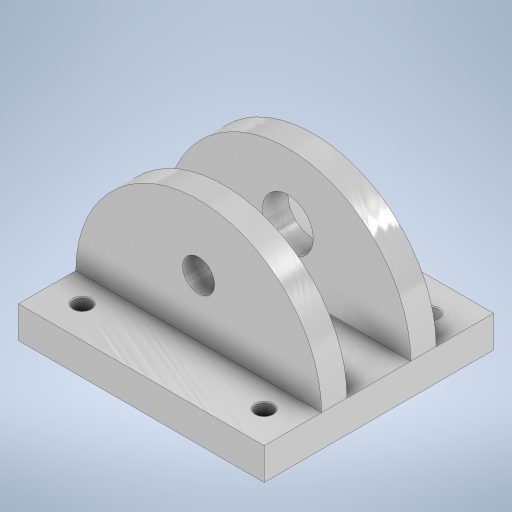
# Autodesk Inventor part: Carriage Top
Saved by Autodesk Inventor 2023 (Build 270158000, 158)
## iProperties
Created: 2023-02-13
Part Number: Carriage Top
Material: Aluminum 6061
Document SubType Name: Modeling
Designer: mbear
Density: 2.7 g/cm^3
Appearance: Machined - Aluminum
Author: mbear
Autodesk Inventor part; units mm, degrees
ref_plane "YZ Plane" through (0, 0, 0) normal (1, 0, 0) x (0, 1, 0)
sketch "Sketch1" plane through (0, 0, 0) normal (0, 1, 0) x (-1, 0, 0)
  line L0 (0, 0) -> (-48.9966, 0)
  line L1 (-48.9966, 0) -> (-48.9966, -45.72)
  line L2 (-48.9966, -45.72) -> (0, -45.72)
  line L3 (0, -45.72) -> (0, 0)
  dimension "d0" = 48.9966
  dimension "d1" = 45.72
  constraints: 8 end point, 2 parallel, 1 horizontal, 1 perpendicular
  measures "d0" distance between parallel lines of L1 L3
  measures "d1" distance between parallel lines of L0 L2
extrude "Extrusion1" add sketch "Sketch1" along normal blind 6.35
sketch "Sketch3" plane through (0, 6.35, 0) normal (0, 1, 0) x (1, 0, 0)
  line L0 (0, 45.72) -> (0, 0) projected
  line L1 (48.9966, 0) -> (48.9966, 45.72) projected
  line L2 (0, 29.21) -> (48.9966, 29.21)
  line L3 (48.9966, 29.21) -> (48.9966, 16.51)
  line L4 (48.9966, 16.51) -> (0, 16.51)
  line L5 (0, 16.51) -> (0, 29.21)
  line L6 (48.9966, 45.72) -> (0, 45.72) projected
  dimension "d4" = 12.7
  dimension "d5" = 16.51
  constraints: 8 end point, 2 parallel, 2 point on line, 1 horizontal, 1 perpendicular
  measures "d4" distance between parallel lines of L4 L2
  measures "d5" distance between parallel lines of L2 L6
sketch "Sketch4" plane through (0, 6.35, 0) normal (0, 1, 0) x (1, 0, 0)
  circle A0 centre (6.35, 39.37) radius 2.1364
  circle A1 centre (42.6466, 39.37) radius 3.0733
  line L0 (48.9966, 45.72) -> (0, 45.72) projected
  line L1 (48.9966, 0) -> (48.9966, 45.72) projected
  line L2 (0, 45.72) -> (0, 0) projected
  circle A2 centre (6.35, 6.35) radius 2.2799
  circle A3 centre (42.6466, 6.35) radius 1.194
  line L3 (0, 0) -> (48.9966, 0) projected
  dimension "d6" = 6.1465
  dimension "d7" = 6.35
  dimension "d8" = 6.35
  dimension "d9" = 6.35
  dimension "d10" = 6.35
  dimension "d11" = 6.35
  dimension "d12" = 6.35
  dimension "d13" = 6.35
  dimension "d14" = 6.35
  constraints: 4 centre point
  measures "d6" diameter of A1
  measures "d7" distance from line of L0 A1.centre
  measures "d8" distance from line of L1 A1.centre
  measures "d9" distance from line of L2 A0.centre
  measures "d10" distance from line of L0 A0.centre
  measures "d11" distance from line of L2 A2.centre
  measures "d12" distance from line of L3 A2.centre
  measures "d13" distance from line of L3 A3.centre
  measures "d14" distance from line of L1 A3.centre
hole "Hole1" at (6.35, 6.35, -39.37) at (42.6466, 6.35, -39.37) at (42.6466, 6.35, -6.35) at (6.35, 6.35, -6.35) direction (0, -1, 0) diameter 3.4 depth 10 tip angle 118 clearance for "Socket Head Cap Screw" size "M3" standard "Ansi Metric M Profile"
fillet "Fillet1" radius 0.2 4 edges at (42.6466, 6.35, -41.07) (6.35, 6.35, -41.07) (42.6466, 6.35, -8.05) (6.35, 6.35, -8.05)
ref_plane "Work Plane1" through (0, 0, -16.51) normal (0, 0, 1) x (1, 0, 0)
sketch "Sketch5" plane through (0, 0, -16.51) normal (0, 0, 1) x (1, 0, 0)
  line L0 (0, 6.35) -> (48.9966, 6.35)
  line L1 (48.9966, 6.35) -> (0, 6.35) projected
  arc A0 (48.9966, 6.35) -> (0, 6.35) centre (24.4983, 6.35) ccw
  point P0 (0, 0)
  constraints: 2 end point, 2 point on circle, 1 centre point, 1 coincident, 1 midpoint
extrude "Extrusion2" add sketch "Sketch5" along normal blind 5.08
ref_plane "Work Plane2" through (0, 0, -22.86) normal (0, 0, 1) x (1, 0, 0)
mirror "Mirror1" about plane through (0, 0, -22.86) normal (0, 0, 1) of "Extrusion2"
sketch "Sketch6" plane through (0, 0, -11.43) normal (0, 0, 1) x (1, 0, 0)
  circle A0 centre (24.4983, 17.78) radius 3.175
  line L0 (0, 6.35) -> (48.9966, 6.35) projected
  point P0 (0, 0)
  point P1 (24.4983, 6.35)
  point P2 (24.4983, 6.35)
  dimension "d27" = 11.43
  dimension "d28" = 6.35
  constraints: 2 midpoint, 1 centre point, 1 vertical alignment
  measures "d27" distance of point (24.498, 6.35) A0.centre
  measures "d28" diameter of A0
extrude "Extrusion3" cut sketch "Sketch6" against normal up to surface (5.08 mm away)
sketch "Sketch8" plane through (24.4983, 6.35, -29.21) normal (0, 0, 1) x (1, 0, 0)
  circle A0 centre (0, 11.43) radius 3.175 projected
  circle A1 centre (0, 11.43) radius 5.08
  point P0 (-24.4983, -6.35)
  dimension "d34" = 10.16
  constraints: 1 centre point, 1 coincident
  measures "d34" diameter of A1
extrude "Extrusion5" cut sketch "Sketch8" against normal blind 25.4 contours A0 | A1
body "Solid1"
